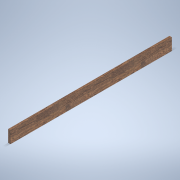
# Autodesk Inventor part: feeding tank bracket
Saved by Autodesk Inventor 2020 (Build 240168000, 168)
## iProperties
Created: 2020-08-16
Part Number: feeding tank bracket
Material: Generic
Document SubType Name: Modeling
Designer: Abbas
Density: 1 g/cm^3
Appearance: Default
Author: Abbas
Autodesk Inventor part; units mm, degrees
ref_plane "YZ Plane" through (0, 0, 0) normal (1, 0, 0) x (0, 1, 0)
ref_plane "XZ Plane" through (0, 0, 0) normal (0, 1, 0) x (-1, 0, 0)
ref_plane "XY Plane" through (0, 0, 0) normal (0, 0, 1) x (1, 0, 0)
sketch "Sketch1" plane through (0, 0, 0) normal (1, 0, 0) x (0, 1, 0)
  line L0 (50, 674) -> (-50, 674)
  line L1 (-50, 674) -> (-50, -674)
  line L2 (-50, -674) -> (50, -674)
  line L3 (50, -674) -> (50, 674)
  line L4 (50, 674) -> (-50, -674) construction
  line L5 (-50, 674) -> (50, -674) construction
  line L6 (50, 0) -> (-50, 0)
  circle A0 centre (25, 654) radius 4
  circle A1 centre (-25, 654) radius 4
  circle A2 centre (25, -654) radius 4
  circle A3 centre (-25, -654) radius 4
  point P0 (0, 0)
  dimension "d0" = 100
  dimension "d1" = 1348
  dimension "d8" = 8
  dimension "d9" = 8
  dimension "d10" = 50
  dimension "d11" = 25
  dimension "d12" = 20
  constraints: 14 end point, 4 centre point, 4 midpoint, 2 parallel, 2 symmetric about line, 1 horizontal, 1 perpendicular, 2 other
  measures "d0" distance of L2.end L1.end
  measures "d1" distance of L1.end L0.end
  measures "d8" diameter of A0
  measures "d9" diameter of A1
  measures "d10" distance of A1.centre A0.centre
  measures "d11" distance from line of L3 A0.centre
  measures "d12" distance from line of L0 A0.centre
extrude "Extrusion2" add sketch "Sketch1" along normal blind 20
sketch "Sketch3" plane through (20, 0, 0) normal (1, 0, 0) x (0, 0, -1)
  line L0 (-200, 25) -> (200, 25)
  line L1 (200, 25) -> (200, -25)
  line L2 (200, -25) -> (-200, -25)
  line L3 (-200, -25) -> (-200, 25)
  circle A0 centre (-200, 25) radius 3
  circle A1 centre (-200, -25) radius 3
  circle A2 centre (200, 25) radius 3
  circle A3 centre (200, -25) radius 3
  line L4 (674, 50) -> (-674, 50) projected
  point P0 (0, 0)
  dimension "d24" = 50
  dimension "d25" = 6
  dimension "d26" = 6
  dimension "d27" = 6
  dimension "d28" = 6
  dimension "d31" = 25
  constraints: 8 end point, 4 centre point, 4 coincident, 2 parallel, 1 horizontal, 1 perpendicular
  measures "d24" distance of L0.end L1.end
  measures "d25" diameter of A0
  measures "d26" diameter of A1
  measures "d27" diameter of A2
  measures "d28" diameter of A3
  measures "d31" distance between parallel lines of L4 L0
extrude "Extrusion4" cut sketch "Sketch3" against normal blind 50 contours L3 A0 L0 | L0 A0 L3 | A2 L1 L0 | L0 L1 A2 | A1 L2 L3 | L3 L2 A1 | A3 L2 L1 | L1 L2 A3
body "Solid2"
